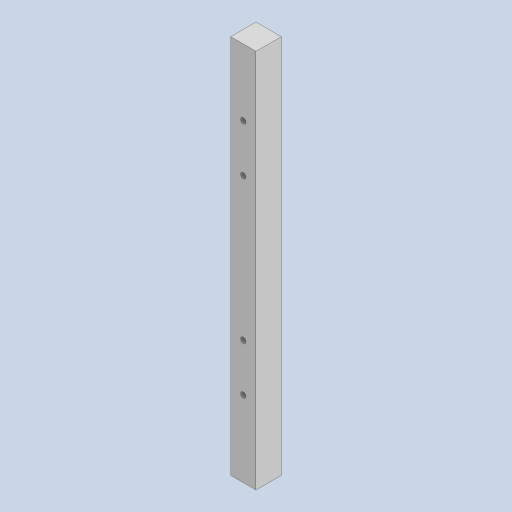
# Autodesk Inventor part: Shorter side frame
Saved by Autodesk Inventor 2023.4 (Build 274418000, 418)
## iProperties
Created: 2024-02-06
Part Number: Shorter side frame
Material: Generic
Document SubType Name: Modeling
Designer: PalumaCMM
Density: 1 g/cm^3
Appearance: Default
Author: PalumaCMM
Autodesk Inventor part; units mm, degrees
ref_plane "YZ Plane" through (0, 0, 0) normal (1, 0, 0) x (0, 1, 0)
ref_plane "XZ Plane" through (0, 0, 0) normal (0, 1, 0) x (-1, 0, 0)
ref_plane "XY Plane" through (0, 0, 0) normal (0, 0, 1) x (1, 0, 0)
sketch "Sketch1" plane through (0, 0, 0) normal (0, 0, 1) x (1, 0, 0)
  line L0 (0, 0) -> (40, 0)
  line L1 (40, 0) -> (40, 600)
  line L2 (40, 600) -> (0, 600)
  line L3 (0, 600) -> (0, 0)
  point P0 (20, 600)
  dimension "d0" = 40
  dimension "d1" = 600
  constraints: 8 end point, 2 parallel, 1 horizontal, 1 midpoint, 1 perpendicular
  measures "d0" distance of L2.end L1.end
  measures "d1" distance of L1.end L0.end
extrude "Extrusion1" add sketch "Sketch1" against normal blind 40
sketch "Sketch2" plane through (0, 0, 0) normal (0, 0, 1) x (1, 0, 0)
  line L0 (40, 600) -> (0, 600) projected
  line L1 (0, 600) -> (0, 0) projected
  line L2 (40, 0) -> (40, 600) projected
  line L3 (0, 0) -> (40, 0) projected
  point P0 (20, 495)
  point P1 (20, 420)
  point P2 (20, 345)
  point P3 (20, 270)
  point P4 (20, 195)
  point P5 (20, 120)
  point P6 (20, 0)
  dimension "d26" = 105
  dimension "d27" = 20
  dimension "d28" = 40
  dimension "d29" = 600
  dimension "d30" = 75
  dimension "d31" = 20
  dimension "d32" = 75
  dimension "d33" = 20
  dimension "d34" = 75
  dimension "d35" = 20
  dimension "d36" = 75
  dimension "d37" = 20
  dimension "d38" = 75
  dimension "d39" = 20
  constraints: 1 midpoint
  measures "d26" distance from line of L0 point (20, 495)
  measures "d27" distance from line of L1 point (20, 495)
  measures "d28" distance between parallel lines of L2 L1
  measures "d29" distance from line of point (20, 0) L0
  measures "d30" distance of point (20, 495) point (20, 420)
  measures "d31" distance from line of L1 point (20, 420)
  measures "d32" distance of point (20, 420) point (20, 345)
  measures "d33" distance from line of L1 point (20, 345)
  measures "d34" distance of point (20, 345) point (20, 270)
  measures "d35" distance from line of L1 point (20, 270)
  measures "d36" distance of point (20, 270) point (20, 195)
  measures "d37" distance from line of L1 point (20, 195)
  measures "d38" distance of point (20, 195) point (20, 120)
  measures "d39" distance from line of L1 point (20, 120)
hole "Hole1" at (20, 495, 0) at (20, 420, 0) at (20, 195, 0) at (20, 120, 0) direction (0, 0, -1) diameter 8.376 end through all thread size "M10x1.5" class "6H" standard "ISO Metric profile"
equation "\"d27\" = 0.5 * d28"
equation "\"d31\" = d27"
equation "\"d32\" = d30"
equation "\"d33\" = d31"
equation "\"d34\" = d32"
equation "\"d35\" = d33"
equation "\"d36\" = d34"
equation "\"d37\" = d35"
equation "\"d38\" = d36"
equation "\"d39\" = d37"
body "Solid1"
